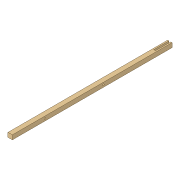
# Autodesk Inventor part: tailboom
Saved by Autodesk Inventor 2019 (Build 230136000, 136)
## iProperties
Created: 2022-04-02
Part Number: tailboom
Material: Balsa
Document SubType Name: Modeling
Designer: solyo
Density: 0.166079 g/cm^3
Appearance: Default(1)
Mass: 10.0542 g
Surface Area: 222.473 cm^2
Volume: 60.5384 cm^3
Author: solyo
Autodesk Inventor part; units mm, degrees
ref_plane "YZ Plane" through (0, 0, 0) normal (1, 0, 0) x (0, 1, 0)
ref_plane "XZ Plane" through (0, 0, 0) normal (0, 1, 0) x (-1, 0, 0)
ref_plane "XY Plane" through (0, 0, 0) normal (0, 0, 1) x (1, 0, 0)
sketch "Sketch1" plane through (0, 0, 0) normal (0, 0, 1) x (1, 0, 0)
  line L0 (-6, -6) -> (6, -6)
  line L1 (6, -6) -> (6, 6)
  line L2 (6, 6) -> (-6, 6)
  line L3 (-6, 6) -> (-6, -6)
  line L4 (-6, -6) -> (6, 6) construction
  line L5 (6, -6) -> (-6, 6) construction
  point P0 (0, 0)
  dimension "d0" = 12
  dimension "d1" = 12
  constraints: 12 end point, 2 midpoint, 2 parallel, 1 horizontal, 1 perpendicular
  measures "d0" distance of L2.end L1.end
  measures "d1" distance of L1.end L0.end
extrude "Extrusion1" add sketch "Sketch1" along normal blind 440
sketch "Sketch4" plane through (-6, 6, 0) normal (0, 1, 0) x (1, 0, 0)
  line L0 (12, 0) -> (0, 0) projected
  line L1 (0, 0) -> (0, -440) projected
  line L2 (12, -440) -> (0, -440) projected
  line L3 (12, 0) -> (12, -440) projected
  line L4 (3.5, 0) -> (3.5, -42)
  line L5 (3.5, -42) -> (8.5, -42)
  line L6 (8.5, -42) -> (8.5, 0)
  point P0 (6, 0)
  point P1 (6, -42)
  point P2 (6, 0)
  dimension "d17" = 5
  dimension "d18" = 42
  constraints: 6 end point, 2 midpoint, 2 perpendicular, 2 point on line, 1 parallel, 1 vertical alignment
  measures "d17" distance of L4.end L5.end
  measures "d18" distance of L5.end L6.end
extrude "Extrusion3" cut sketch "Sketch4" against normal through all contours L6 L5 L4 L0
sketch "Sketch5" plane through (6, -6, 0) normal (1, 0, 0) x (0, 0, -1)
  line L0 (-440, 0) -> (-440, 12) projected
  point P0 (0, 6)
  point P1 (-350, 6)
  point P2 (-189, 6)
  point P3 (-440, 6)
  dimension "d21" = 161
  dimension "d24" = 90
  constraints: 2 horizontal alignment, 1 midpoint
  measures "d21" distance of point (-189, 6) point (-350, 6)
  measures "d24" distance of point (-440, 6) point (-350, 6)
hole "Hole2" at (6, 0, 350) at (6, 0, 189) direction (-1, 0, 0) diameter 4 end through all
equation "\"d0\" = d1"
body "Solid1"
